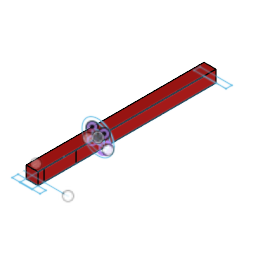
Puncher (Autodesk Fusion 360 design; units mm, degrees)
part number: 2026-05-29-18-08-39-513
Autodesk Fusion 360 part; units mm, degrees
sketch "Sketch1" plane through (0, 0, 0) normal (0, 0, 1) x (1, 0, 0)
  line L0 (99, -7) -> (99, 28)
  line L1 (96, 28) -> (96, -7)
  line L2 (96, -18) -> (96, -7)
  line L3 (99, -18) -> (96, -18)
  line L4 (99, -15) -> (99, -18)
  line L5 (101, -18) -> (94, -18)
  line L6 (94, -16.5) -> (101, -16.5)
  line L7 (101, -16.5) -> (101, -18)
  line L8 (94, -18) -> (94, -16.5)
  line L9 (95, 0) -> (100, 0)
  line L10 (94, -15) -> (105, -15)
  line L11 (94, -16.5) -> (94, -12) construction
  line L12 (99, -7) -> (99, -15)
  line L13 (96, 28) -> (99, 28)
  line L14 (97.5, 28) -> (101.5, 28) construction
  line L15 (101.5, 28) -> (93.5, 28)
  line L16 (93.5, 28) -> (93.5, 29.5)
  line L17 (93.5, 29.5) -> (101.5, 29.5)
  line L18 (101.5, 29.5) -> (101.5, 28)
  dimension "d1" = 5
  dimension "d2" = 3
  dimension "d6" = 7
  dimension "d7" = 1.5
  dimension "d10" = 4
  dimension "d11" = 8
  dimension "d12" = 1.5
  dimension "d18" = 43
  dimension "d19" = 28
  dimension "d26" = 16.5
  constraint horizontal L9
  constraint vertical L0
  constraint vertical L1
  constraint vertical L4
  constraint horizontal L3
  constraint vertical L2
  constraint horizontal L6
  constraint vertical L7
  constraint horizontal L5
  constraint vertical L8
  constraint perpendicular L10 L11
  constraint coincident L11 L10.start
  constraint perpendicular L0 L13
  constraint midpoint L13 L14.start
  constraint perpendicular L1 L14
  constraint horizontal L15
  constraint vertical L16
  constraint horizontal L17
  constraint vertical L18
  measures "d1" distance of L9.start L9.end
  measures "d2" distance of L1.end L0.start
  measures "d6" distance of L6.end L6.start
  measures "d7" distance of L6.start L5.end
  measures "d10" distance of L14.start L14.end
  measures "d11" distance of L14.end L15.end
  measures "d12" distance of L14.end L17.end
  measures "d18" distance of L10 L13
  measures "d19" distance of L9 L14
  measures "d26" distance of L6 L9
extrude "Extrude4" add sketch "Sketch1" along normal blind 3 contours L0 L1 L2 L9 L10 L12 | L0 L1 L9 L13 L15 | L2 L4 L6 L10
sketch "Sketch3" plane through (0, 0, 0) normal (0, 1, 0) x (1, 0, 0)
  line L0 (96, -3) -> (99, -3)
  line L1 (96, 0) -> (96, -3)
  line L2 (99, 0) -> (99, -3)
  line L3 (99, 0) -> (96, 0)
  line L4 (97.5, 0) -> (97.5, -1.5) construction
  circle A0 centre (97.5, -1.5) radius 1.5
  circle A1 centre (97.5, -1.5) radius 4
  circle A2 centre (97.5, -1.5) radius 3
  line L5 (97.5, -1.5) -> (98, -1.5) construction
  line L6 (98, -1.5) -> (98, -1) construction
  line L7 (98, -1) -> (97, -1)
  line L8 (97, -1) -> (97, -2)
  line L9 (97, -2) -> (98, -2)
  line L10 (98, -2) -> (98, -1)
  line L11 (97, -2) -> (96.3, -2)
  line L12 (96.3, -2) -> (96.3, -1)
  line L13 (96.3, -1) -> (97, -1)
  line L14 (97, -1) -> (97, -2)
  line L15 (97, -1) -> (98, -1)
  line L16 (98, -1) -> (98, -0.3)
  line L17 (98, -0.3) -> (97, -0.3)
  line L18 (97, -0.3) -> (97, -1)
  line L19 (98, -1) -> (98.7, -1)
  line L20 (98.7, -1) -> (98.7, -2)
  line L21 (98.7, -2) -> (98, -2)
  line L22 (98, -2) -> (98, -1)
  line L23 (97, -2) -> (98, -2)
  line L24 (98, -2) -> (98, -2.7)
  line L25 (98, -2.7) -> (97, -2.7)
  line L26 (97, -2.7) -> (97, -2)
  constraint midpoint L3 L4.start
  constraint perpendicular L3 L4
  constraint coincident L4.end A0.centre
  constraint tangent L2 A0
  constraint concentric A0 A1
  constraint perpendicular L4 L5
  constraint perpendicular L5 L6
  constraint horizontal L7
  constraint vertical L8
  constraint horizontal L9
  constraint vertical L10
  constraint horizontal L11
  constraint vertical L12
  constraint horizontal L13
  constraint vertical L14
  constraint horizontal L15
  constraint vertical L16
  constraint horizontal L17
  constraint vertical L18
  constraint horizontal L19
  constraint vertical L20
  constraint horizontal L21
  constraint vertical L22
  constraint horizontal L23
  constraint vertical L24
  constraint horizontal L25
  constraint vertical L26
extrude "Extrude5" [suppressed]
extrude "Extrude6" [suppressed]
extrude "Extrude7" [suppressed]
extrude "Extrude8" [suppressed]
extrude "Extrude9" [suppressed]
extrude "Extrude10" [suppressed]
extrude "Extrude11" [suppressed]
move_body "Move1" [suppressed]
move_body "Move2" [suppressed]
coilprimitive "CoilPrimitive1" [suppressed]
extrude "Extrude1" [suppressed]
sketch "Sketch2" plane through (0, 0, 0) normal (0, 1, 0) x (1, 0, 0)
  line L0 (96, -3) -> (99, -3)
  line L1 (96, 0) -> (96, -3)
  line L2 (99, 0) -> (99, -3)
  line L3 (94, 0) -> (105, 0)
  line L4 (97.5, -3) -> (97.5, 0) construction
  line L5 (99, -1.5) -> (96, -1.5) construction
  circle A0 centre (97.5, -1.5) radius 4
  circle A1 centre (97.5, -1.5) radius 1.5
  line L6 (97.5, -1.5) -> (98, -1.5) construction
  line L7 (98, -1.5) -> (98, -2) construction
  line L8 (98, -2) -> (97, -2)
  line L9 (97, -2) -> (97, -1)
  line L10 (97, -1) -> (98, -1)
  line L11 (98, -1) -> (98, -2)
  line L12 (97, -1.5) -> (97, -1.75) construction
  line L13 (97, -2) -> (96.5, -2)
  line L14 (96.5, -2) -> (96.5, -1)
  line L15 (96.5, -1) -> (97, -1)
  line L16 (97, -1) -> (97, -2)
  line L17 (97, -2.5) -> (97, -2)
  line L18 (98, -2.5) -> (97, -2.5)
  line L19 (98, -2) -> (98, -2.5)
  line L20 (98.5, -2) -> (98, -2)
  line L21 (98.5, -1) -> (98.5, -2)
  line L22 (98, -1) -> (98.5, -1)
  line L23 (98, -0.5) -> (98, -1)
  line L24 (97, -0.5) -> (98, -0.5)
  line L25 (97, -1) -> (97, -0.5)
  dimension "d13" = 8
  dimension "d23" = 0.25
  dimension "d25" = 360
  constraint midpoint L0 L4.start
  constraint coincident L3 L4.end
  constraint perpendicular L3 L4
  constraint midpoint L2 L5.start
  constraint midpoint L1 L5.end
  constraint midpoint L5 A0.centre
  constraint concentric A0 A1
  constraint coincident L5.start A1
  constraint coincident A0.centre A1.centre
  constraint coincident L5 L6.end
  constraint perpendicular L5 L7
  constraint horizontal L8
  constraint vertical L9
  constraint horizontal L10
  constraint vertical L11
  constraint midpoint L9 L12.start
  constraint perpendicular L5 L12
  constraint horizontal L13
  constraint vertical L14
  constraint horizontal L15
  constraint vertical L16
  measures "d13" diameter of A0
  measures "d23" distance of L12.start L12.end
extrude "Extrude2" [suppressed]
extrude "Extrude3" [suppressed]
